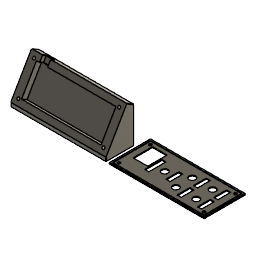
SoundRat (Autodesk Fusion 360 design; units mm, degrees)
Autodesk Fusion 360 part; units mm, degrees
sketch "Sketch1" plane through (0, 0, 0) normal (0, 0, 1) x (1, 0, 0)
  line L0 (74.95, -104) -> (175, -104)
  line L1 (175, -104) -> (175, -141.6)
  line L2 (175, -141.6) -> (74.95, -141.6)
  line L3 (74.95, -141.6) -> (74.95, -104)
  line L4 (67.45, -96.5) -> (182.5, -96.5)
  line L5 (182.5, -96.5) -> (182.5, -149.1)
  line L6 (182.5, -149.1) -> (67.45, -149.1)
  line L7 (67.45, -149.1) -> (67.45, -96.5)
  line L8 (67.45, -99) -> (64.95, -99)
  line L9 (64.95, -99) -> (64.95, -146.6)
  line L10 (64.95, -146.6) -> (67.45, -146.6)
  line L11 (67.45, -146.6) -> (67.45, -99)
  line L12 (182.5, -99) -> (185, -99)
  line L13 (185, -99) -> (185, -146.6)
  line L14 (185, -146.6) -> (182.5, -146.6)
  line L15 (182.5, -146.6) -> (182.5, -99)
  line L16 (78.95, -104) -> (88.95, -104)
  line L17 (88.95, -104) -> (88.95, -96.5)
  line L18 (88.95, -96.5) -> (78.95, -96.5)
  line L19 (78.95, -96.5) -> (78.95, -104)
  circle A0 centre (71.45, -103) radius 1.7
  circle A1 centre (71.45, -103) radius 3
  circle A2 centre (71.45, -142.6) radius 3
  circle A3 centre (71.45, -142.6) radius 1.7
  circle A4 centre (178.5, -103) radius 3
  circle A5 centre (178.5, -103) radius 1.7
  circle A6 centre (178.5, -142.6) radius 3
  circle A7 centre (178.5, -142.6) radius 1.7
  line L20 (182.5, -149.1) -> (185, -149.1)
  line L21 (185, -149.1) -> (185, -146.6)
  line L22 (185, -146.6) -> (182.5, -146.6)
  line L23 (182.5, -146.6) -> (182.5, -149.1)
  line L24 (185, -99) -> (182.5, -99)
  line L25 (182.5, -99) -> (182.5, -96.5)
  line L26 (182.5, -96.5) -> (185, -96.5)
  line L27 (185, -96.5) -> (185, -99)
  line L28 (67.45, -96.5) -> (64.95, -96.5)
  line L29 (64.95, -96.5) -> (64.95, -99)
  line L30 (64.95, -99) -> (67.45, -99)
  line L31 (67.45, -99) -> (67.45, -96.5)
  line L32 (67.45, -149.1) -> (64.95, -149.1)
  line L33 (64.95, -149.1) -> (64.95, -146.6)
  line L34 (64.95, -146.6) -> (67.45, -146.6)
  line L35 (67.45, -146.6) -> (67.45, -149.1)
  dimension "d1" = 100.05
  dimension "d2" = 37.6
  dimension "d3" = 7.5
  dimension "d4" = 7.5
  dimension "d5" = 7.5
  dimension "d6" = 7.5
  dimension "d7" = 2.5
  dimension "d8" = 2.5
  dimension "d9" = 2.5
  dimension "d10" = 2.5
  dimension "d11" = 2.5
  dimension "d12" = 2.5
  dimension "d19" = 4
  dimension "d20" = 10
  dimension "d26" = 3.4
  dimension "d29" = 6.5
  dimension "d30" = 4
  dimension "d31" = 6
  dimension "d32" = 3.4
  dimension "d33" = 6
  dimension "d34" = 6.5
  dimension "d35" = 4
  dimension "d36" = 3.4
  dimension "d37" = 6
  dimension "d38" = 3.4
  dimension "d39" = 6
  dimension "d40" = 6.5
  dimension "d41" = 4
  dimension "d42" = 4
  dimension "d43" = 6.5
  constraint horizontal L0
  constraint vertical L1
  constraint horizontal L2
  constraint vertical L3
  constraint horizontal L4
  constraint vertical L5
  constraint horizontal L6
  constraint vertical L7
  constraint horizontal L8
  constraint vertical L9
  constraint horizontal L10
  constraint vertical L11
  constraint coincident L7 L8.start
  constraint horizontal L12
  constraint vertical L13
  constraint horizontal L14
  constraint vertical L15
  constraint coincident L5 L12.start
  constraint horizontal L16
  constraint vertical L17
  constraint horizontal L18
  constraint vertical L19
  constraint coincident L4 L17.end
  constraint coincident L0 L16.start
  constraint concentric A0 A1
  constraint concentric A2 A3
  constraint concentric A4 A5
  constraint concentric A6 A7
  constraint horizontal L20
  constraint vertical L21
  constraint horizontal L22
  constraint vertical L23
  constraint horizontal L24
  constraint vertical L25
  constraint horizontal L26
  constraint vertical L27
  constraint horizontal L28
  constraint vertical L29
  constraint horizontal L30
  constraint vertical L31
  constraint horizontal L32
  constraint vertical L33
  constraint horizontal L34
  constraint vertical L35
  measures "d1" distance of L1 L3
  measures "d2" distance of L0 L2
  measures "d3" distance of L0 L4
  measures "d4" distance of L1 L5
  measures "d5" distance of L3 L7
  measures "d6" distance of L2 L6
  measures "d7" distance of L4 L8
  measures "d8" distance of L6 L10
  measures "d9" distance of L9 L11
  measures "d10" distance of L6 L14
  measures "d11" distance of L4 L12
  measures "d12" distance of L13 L15
  measures "d19" distance of L3 L19
  measures "d20" distance of L17 L19
  measures "d26" diameter of A0
  measures "d29" distance of L4 A0.centre
  measures "d30" distance of L7 A0.centre
  measures "d31" diameter of A1
  measures "d32" diameter of A3
  measures "d33" diameter of A2
  measures "d34" distance of L6 A2.centre
  measures "d35" distance of L7 A2.centre
  measures "d36" diameter of A5
  measures "d37" diameter of A4
  measures "d38" diameter of A7
  measures "d39" diameter of A6
  measures "d40" distance of L4 A4.centre
  measures "d41" distance of L15 A4.centre
  measures "d42" distance of L15 A6.centre
  measures "d43" distance of L6 A6.centre
sketch "Sketch3" plane through (0, 0, 0) normal (0, 0, 1) x (1, 0, 0)
  line L0 (181.1, -169) -> (183.6, -169)
  line L1 (181.1, -219.1) -> (66.05, -219.1)
  circle A0 centre (70.05, -212.6) radius 1.7
  line L2 (183.6, -169) -> (183.6, -216.6)
  line L3 (181.1, -166.5) -> (181.1, -219.1)
  line L4 (63.55, -216.6) -> (66.05, -216.6)
  line L5 (66.05, -216.6) -> (66.05, -169)
  line L6 (66.05, -219.1) -> (66.05, -166.5)
  line L7 (73.55, -174) -> (173.6, -174)
  line L8 (183.6, -216.6) -> (181.1, -216.6)
  line L9 (181.1, -216.6) -> (181.1, -169)
  circle A1 centre (70.05, -173) radius 1.7
  line L10 (63.55, -169) -> (63.55, -216.6)
  circle A2 centre (177.1, -173) radius 1.7
  circle A3 centre (177.1, -212.6) radius 1.7
  line L11 (88.45, -166.5) -> (79.45, -166.5)
  line L12 (73.55, -211.6) -> (73.55, -174)
  line L13 (173.6, -174) -> (173.6, -211.6)
  line L14 (66.05, -169) -> (63.55, -169)
  line L15 (66.05, -166.5) -> (181.1, -166.5)
  line L16 (173.6, -211.6) -> (73.55, -211.6)
  line L17 (79.45, -174) -> (88.45, -174)
  line L18 (93.5, -182.12) -> (98.5, -182.12)
  line L19 (98.5, -182.12) -> (98.5, -203.52)
  line L20 (98.5, -203.52) -> (93.5, -203.52)
  line L21 (93.5, -203.52) -> (93.5, -182.12)
  circle A4 centre (108.1, -193.12) radius 4
  line L22 (117.45, -184.87) -> (122.45, -184.87)
  line L23 (122.45, -184.87) -> (122.45, -200.77)
  line L24 (122.45, -200.77) -> (117.45, -200.77)
  line L25 (117.45, -200.77) -> (117.45, -184.87)
  circle A5 centre (132.45, -182.76) radius 4
  circle A6 centre (132.45, -203.45) radius 4
  line L26 (141.75, -174.5) -> (146.75, -174.5)
  line L27 (141.75, -190.5) -> (141.75, -174.5)
  line L28 (146.75, -190.5) -> (141.75, -190.5)
  line L29 (146.75, -174.5) -> (146.75, -190.5)
  line L30 (146.75, -195.1) -> (146.75, -211.1)
  line L31 (146.75, -211.1) -> (141.75, -211.1)
  line L32 (141.75, -211.1) -> (141.75, -195.1)
  line L33 (141.75, -195.1) -> (146.75, -195.1)
  circle A7 centre (158.1, -182.76) radius 4
  circle A8 centre (158.1, -203.45) radius 4
  line L34 (167.4, -211.1) -> (167.4, -195.1)
  line L35 (167.4, -195.1) -> (172.4, -195.1)
  line L36 (172.4, -195.1) -> (172.4, -211.1)
  line L37 (172.4, -211.1) -> (167.4, -211.1)
  line L38 (172.4, -190.5) -> (167.4, -190.5)
  line L39 (172.4, -174.5) -> (172.4, -190.5)
  line L40 (167.4, -174.5) -> (172.4, -174.5)
  line L41 (167.4, -190.5) -> (167.4, -174.5)
  line L42 (66.05, -169) -> (181.1, -169)
  line L43 (66.05, -216.6) -> (181.1, -216.6)
  line L44 (183.6, -169) -> (181.1, -169)
  line L45 (181.1, -169) -> (181.1, -166.5)
  line L46 (181.1, -166.5) -> (183.6, -166.5)
  line L47 (183.6, -166.5) -> (183.6, -169)
  line L48 (183.6, -216.6) -> (181.1, -216.6)
  line L49 (181.1, -216.6) -> (181.1, -219.1)
  line L50 (181.1, -219.1) -> (183.6, -219.1)
  line L51 (183.6, -219.1) -> (183.6, -216.6)
  line L52 (66.05, -219.1) -> (63.55, -219.1)
  line L53 (63.55, -219.1) -> (63.55, -216.6)
  line L54 (63.55, -216.6) -> (66.05, -216.6)
  line L55 (66.05, -216.6) -> (66.05, -219.1)
  line L56 (63.55, -169) -> (66.05, -169)
  line L57 (66.05, -169) -> (66.05, -166.5)
  line L58 (66.05, -166.5) -> (63.55, -166.5)
  line L59 (63.55, -166.5) -> (63.55, -169)
  dimension "d48" = 100.05
  dimension "d49" = 37.6
  dimension "d50" = 7.5
  dimension "d51" = 7.5
  dimension "d52" = 7.5
  dimension "d53" = 7.5
  dimension "d54" = 2.5
  dimension "d55" = 2.5
  dimension "d56" = 2.5
  dimension "d57" = 2.5
  dimension "d58" = 2.5
  dimension "d59" = 2.5
  dimension "d62" = 3.4
  dimension "d64" = 4
  dimension "d66" = 3.4
  dimension "d69" = 4
  dimension "d70" = 3.4
  dimension "d72" = 3.4
  dimension "d75" = 4
  dimension "d76" = 4
  dimension "d78" = 19.95
  dimension "d79" = 8.12
  dimension "d80" = 8.08
  dimension "d81" = 21.4
  dimension "d82" = 8
  dimension "d83" = 19.12
  dimension "d84" = 34.55
  dimension "d86" = 5
  dimension "d87" = 5
  dimension "d88" = 10.87
  dimension "d89" = 10.83
  dimension "d90" = 15.9
  dimension "d91" = 9.35
  dimension "d92" = 8
  dimension "d93" = 10
  dimension "d94" = 8.76
  dimension "d95" = 8
  dimension "d96" = 10
  dimension "d97" = 20.69
  dimension "d98" = 5
  dimension "d100" = 9.3
  dimension "d101" = 0.5
  dimension "d102" = 16
  dimension "d103" = 5
  dimension "d104" = 16
  dimension "d105" = 0.5
  dimension "d106" = 9.3
  dimension "d107" = 8
  dimension "d108" = 8
  dimension "d109" = 20.69
  dimension "d110" = 5
  dimension "d111" = 9.3
  dimension "d112" = 16
  dimension "d113" = 5
  dimension "d114" = 16
  dimension "d115" = 9.3
  dimension "d116" = 25.65
  dimension "d131" = 4
  dimension "d132" = 4
  dimension "d133" = 4
  dimension "d134" = 4
  constraint horizontal L7
  constraint vertical L13
  constraint horizontal L16
  constraint vertical L12
  constraint horizontal L15
  constraint vertical L3
  constraint horizontal L1
  constraint vertical L6
  constraint horizontal L14
  constraint vertical L10
  constraint horizontal L4
  constraint vertical L5
  constraint coincident L5.end L6
  constraint horizontal L0
  constraint vertical L2
  constraint horizontal L8
  constraint vertical L9
  constraint coincident L0.start L3
  constraint horizontal L17
  constraint horizontal L11
  constraint coincident L11.start L15
  constraint coincident L17.start L7
  constraint horizontal L18
  constraint vertical L19
  constraint horizontal L20
  constraint vertical L21
  constraint horizontal L22
  constraint vertical L23
  constraint horizontal L24
  constraint vertical L25
  constraint horizontal L26
  constraint vertical L29
  constraint horizontal L28
  constraint vertical L27
  constraint horizontal L33
  constraint vertical L30
  constraint horizontal L31
  constraint vertical L32
  constraint horizontal L40
  constraint vertical L39
  constraint horizontal L38
  constraint vertical L41
  constraint horizontal L35
  constraint vertical L36
  constraint horizontal L37
  constraint vertical L34
  constraint horizontal L44
  constraint vertical L45
  constraint horizontal L46
  constraint vertical L47
  constraint horizontal L48
  constraint vertical L49
  constraint horizontal L50
  constraint vertical L51
  constraint horizontal L52
  constraint vertical L53
  constraint horizontal L54
  constraint vertical L55
  constraint horizontal L56
  constraint vertical L57
  constraint horizontal L58
  constraint vertical L59
  measures "d48" distance of L12 L13
  measures "d49" distance of L7 L16
  measures "d50" distance of L7 L15
  measures "d51" distance of L3 L13
  measures "d52" distance of L6 L12
  measures "d53" distance of L1 L16
  measures "d54" distance of L14 L15
  measures "d55" distance of L1 L4
  measures "d56" distance of L5 L10
  measures "d57" distance of L1 L8
  measures "d58" distance of L0 L15
  measures "d59" distance of L2 L9
  measures "d62" diameter of A1
  measures "d64" distance of A1.centre L6
  measures "d66" diameter of A0
  measures "d69" distance of A0.centre L6
  measures "d70" diameter of A2
  measures "d72" diameter of A3
  measures "d75" distance of A2.centre L9
  measures "d76" distance of A3.centre L9
  measures "d78" distance of L12 L21
  measures "d79" distance of L7 L18
  measures "d80" distance of L16 L20
  measures "d81" distance of L18 L20
  measures "d82" diameter of A4
  measures "d83" distance of L7 A4.centre
  measures "d84" distance of L12 A4.centre
  measures "d86" distance of L19 L21
  measures "d87" distance of L23 L25
  measures "d88" distance of L7 L22
  measures "d89" distance of L16 L24
  measures "d90" distance of L22 L24
  measures "d91" distance of A4.centre L25
  measures "d92" diameter of A5
  measures "d93" distance of L23 A5.centre
  measures "d94" distance of L7 A5.centre
  measures "d95" diameter of A6
  measures "d96" distance of L23 A6.centre
  measures "d97" distance of A5.centre A6.centre
  measures "d98" distance of L27 L29
  measures "d100" distance of A5.centre L27
  measures "d101" distance of L7 L26
  measures "d102" distance of L26 L28
  measures "d103" distance of L30 L32
  measures "d104" distance of L31 L33
  measures "d105" distance of L16 L31
  measures "d106" distance of A6.centre L32
  measures "d107" diameter of A7
  measures "d108" diameter of A8
  measures "d109" distance of A8.centre A7.centre
  measures "d110" distance of L39 L41
  measures "d111" distance of A7.centre L41
  measures "d112" distance of L38 L40
  measures "d113" distance of L34 L36
  measures "d114" distance of L35 L37
  measures "d115" distance of A8.centre L34
  measures "d116" distance of A5.centre A7.centre
  measures "d131" distance of A1.centre L42
  measures "d132" distance of A2.centre L42
  measures "d133" distance of A0.centre L43
  measures "d134" distance of A3.centre L43
move_body "Move1" [no effect]
move_body "Move2" [no effect]
move_body "Move3" [no effect]
move_body "Move4" [no effect]
move_body "Move5" [no effect]
extrude "Extrude16" add sketch "Sketch1" along normal blind 2.5 contours L0 L1 L2 L3 L16 makes body 1
extrude "Extrude17" add sketch "Sketch1" along normal blind 10.4 contours L0 L1 L2 L3 L4 L5 L6 L7 L11 L15 L17 L19 L23 L25 L31 L35 | L0 L4 L16 L17 L18 L19 | L7 L8 L28 L29 L30 L31 | L5 L12 L24 L25 L26 L27 | L7 L8 L9 L10 L11 L30 L34 | L5 L12 L13 L14 L15 L22 L24 | L7 L10 L32 L33 L34 L35 | L5 L14 L20 L21 L22 L23 | A0 | A1 | A2 | A3 | A4 | A5 | A6 | A7 bodies 1
extrude "Extrude18" cut sketch "Sketch1" along normal blind 6 from surface at 5 contours L0 L4 L16 L17 L18 L19 bodies 1
extrude "Extrude19" cut sketch "Sketch1" along normal blind 3.1 contours A1 | A2 | A4 | A6 bodies 1
extrude "Extrude20" cut sketch "Sketch1" along normal blind 10.4 contours A0 | A3 | A5 | A7 bodies 1
move_body "Move6" bodies 1 to x (1, 0, 0) y (0, 0.5, 0.866025) z (0, -0.866025, 0.5) at (0, -74.55, 129.1244)
sketch "Sketch7" plane through (64.95, 0, 0) normal (-1, 0, 0) x (0, -1, 0)
  line L0 (122.8, 45.5529) -> (149.1, 0)
  line L1 (149.1, 0) -> (158.1067, 5.2)
  line L2 (158.1067, 5.2) -> (131.8067, 50.7529)
  line L3 (131.8067, 50.7529) -> (122.8, 45.5529)
  line L4 (122.8, 45.5529) -> (122.8, 0)
  line L5 (122.8, 0) -> (149.1, 0)
  line L6 (158.1067, 5.2) -> (158.1067, 0)
  line L7 (158.1067, 0) -> (149.1, 0)
  constraint coincident L0.start L3.end
  constraint vertical L4
  constraint coincident L0.end L1.start
  constraint perpendicular L4 L5
  constraint coincident L1.end L2.start
  constraint vertical L6
  constraint perpendicular L6 L7
extrude "Extrude21" add sketch "Sketch7" against normal blind 120 contours L0 L4 L5 | L1 L6 L7 bodies 1
extrude "Extrude22" add 1 faces at (184.95, -131.5667, 15.1843) along direction (1, 0, 0) blind 0.05 on bodies 1 bodies 1
extrude "Extrude23" add 1 faces at (184.95, -155.1044, 1.7333) along direction (1, 0, 0) blind 0.05 on bodies 1 bodies 1
extrude "Extrude24" cut 4 faces at (177.7558, -125.7844, 40.3837) (179.2219, -145.5844, 6.0891) (71.8404, -126.4322, 39.2618) (72.1281, -145.0948, 6.9373) along direction (0, 0.866025, -0.5) blind 40 on bodies 1 bodies 1
extrude "Extrude26" add sketch "Sketch3" along normal blind 1 separate body contours L3 L5 L6 L9 L42 L43 | A0 | L7 L12 L13 L16 L17 | A1 | A2 | A3 makes body 2
extrude "Extrude27" add sketch "Sketch3" along normal blind 1.2 separate body contours L0 L3 L44 L45 L46 L47 | L3 L6 L11 L15 L42 L45 L57 | L0 L2 L3 L8 L9 L44 L48 | L1 L3 L6 L43 L49 L55 | L6 L14 L56 L57 L58 L59 | L4 L5 L6 L10 L14 L54 L56 | L4 L6 L52 L53 L54 L55 makes body 3
extrude "Extrude28" add sketch "Sketch3" along normal blind 1.2 contours L3 L8 L48 L49 L50 L51 bodies 2 3
extrude "Extrude29" add 1 faces at (104.4, -218.2667, 1.2) along direction (0, 0, 1) blind 0.2 on bodies 2 bodies 2
chamfer "Chamfer4" distance 0.5 angle 45 8 edges at (63.55, -192.8, 1.4) (123.575, -166.5, 1.4) (183.6, -192.8, 1.4) (123.575, -219.1, 1.4) (63.55, -219.1, 0.7) (183.6, -219.1, 0.7) (183.6, -166.5, 0.7) (63.55, -166.5, 0.7) on bodies 2
extrude "Extrude30" cut sketch "Sketch3" along normal blind 2 contours A0 | A1 | A2 | A3 bodies 2
chamfer "Chamfer5" distance 0.5 angle 45 2 edges at (83.95, -127.1301, 48.0529) (83.95, -130.8801, 41.5577) on bodies 1
chamfer "Chamfer6" distance 0.5 angle 45 11 edges at (124.975, -158.1067, 0) (64.95, -158.1067, 2.6) (185, -158.1067, 2.6) (185, -140.4533, 0) (185, -122.8, 22.7765) (124.975, -122.8, 0) (124.975, -122.8, 45.5529) (185, -127.3033, 48.1529) (64.95, -127.3033, 48.1529) (64.95, -122.8, 22.7765) (64.95, -140.4533, 0) on bodies 1
chamfer "Chamfer7" distance 0.5 angle 45 2 edges at (88.95, -129.2519, 49.2779) (78.95, -129.2519, 49.2779) on bodies 1
chamfer "Chamfer8" distance 0.5 angle 45 2 edges at (78.95, -133.0019, 42.7827) (88.95, -133.0019, 42.7827) on bodies 1
move_body "Move7" bodies 2 to x (1, 0, 0) y (0, 0.5, 0.866025) z (0, -0.866025, 0.5) at (1.3343, -48.7637, 195.0311)
move_body "Move8" bodies 2 to x (1, 0, 0) y (0, 1, 0) z (0, 0, 1) at (0.1947, 0.0649, 0.1124)
sketch "Sketch8" plane through (0, -121.8898, 70.3731) normal (0, -0.866025, 0.5) x (1, 0, 0)
  circle A0 centre (71.579, -67.9501) radius 1.7
  circle A1 centre (178.629, -67.9501) radius 1.7
  circle A2 centre (71.579, -28.3501) radius 1.7
  circle A3 centre (178.629, -28.3501) radius 1.7
  circle A4 centre (133.979, -58.8001) radius 4
  line L0 (143.279, -66.4501) -> (143.279, -50.4501)
  line L1 (143.279, -50.4501) -> (148.279, -50.4501)
  line L2 (148.279, -50.4501) -> (148.279, -66.4501)
  line L3 (148.279, -66.4501) -> (143.279, -66.4501)
  line L4 (123.979, -56.1201) -> (118.979, -56.1201)
  line L5 (118.979, -56.1201) -> (118.979, -40.2201)
  line L6 (118.979, -40.2201) -> (123.979, -40.2201)
  line L7 (123.979, -40.2201) -> (123.979, -56.1201)
  circle A5 centre (133.979, -38.1101) radius 4
  line L8 (100.029, -58.8701) -> (95.029, -58.8701)
  line L9 (95.029, -58.8701) -> (95.029, -37.4701)
  line L10 (95.029, -37.4701) -> (100.029, -37.4701)
  line L11 (100.029, -37.4701) -> (100.029, -58.8701)
  line L12 (143.279, -29.8501) -> (148.279, -29.8501)
  line L13 (148.279, -29.8501) -> (148.279, -45.8501)
  line L14 (148.279, -45.8501) -> (143.279, -45.8501)
  line L15 (143.279, -45.8501) -> (143.279, -29.8501)
  circle A6 centre (109.629, -48.4701) radius 4
  line L16 (173.929, -50.4501) -> (173.929, -66.4501)
  line L17 (173.929, -66.4501) -> (168.929, -66.4501)
  line L18 (168.929, -66.4501) -> (168.929, -50.4501)
  line L19 (168.929, -50.4501) -> (173.929, -50.4501)
  circle A7 centre (159.629, -38.1101) radius 4
  circle A8 centre (159.629, -58.8001) radius 4
  line L20 (173.929, -45.8501) -> (168.929, -45.8501)
  line L21 (168.929, -45.8501) -> (168.929, -29.8501)
  line L22 (168.929, -29.8501) -> (173.929, -29.8501)
  line L23 (173.929, -29.8501) -> (173.929, -45.8501)
  line L24 (67.579, -24.3501) -> (67.579, -71.9501)
  line L25 (67.579, -71.9501) -> (182.629, -71.9501)
  line L26 (182.629, -71.9501) -> (182.629, -24.3501)
  line L27 (182.629, -24.3501) -> (67.579, -24.3501)
  line L28 (75.079, -53.5201) -> (93.2419, -53.5201)
  line L29 (93.2419, -53.5201) -> (93.2419, -29.3501)
  line L30 (93.2419, -29.3501) -> (75.079, -29.3501)
  line L31 (75.079, -29.3501) -> (75.079, -53.5201)
  dimension "d176" = 5
  dimension "d177" = 7.5
  constraint horizontal L28
  constraint vertical L29
  constraint horizontal L30
  constraint vertical L31
  measures "d176" distance of L27 L30
  measures "d177" distance of L24 L31
extrude "Extrude31" cut sketch "Sketch8" against normal blind 2 contours L28 L29 L30 L31 bodies 2
move_body "Move9" bodies 2 to x (1, 0, 0) y (0, 0.5, -0.866025) z (0, 0.866025, 0.5) at (124, -84.2799, -135.1823)
move_body "Move10" bodies 2 to x (1, 0, 0) y (0, 1, 0) z (0, 0, 1) at (0, 0, -4)
equation "d1 = 99.95 mm + 0.1 mm"
equation "d2 = 37.5 mm + 0.1 mm"
equation "d29 = 4 mm + 2.5 mm"
equation "d34 = 4 mm + 2.5 mm"
equation "d40 = 4 mm + 2.5 mm"
equation "d43 = 4.00 mm + 2.5 mm"
equation "d48 = 99.95 mm + 0.1 mm"
equation "d49 = 37.5 mm + 0.1 mm"
equation "d78 = 19.85 mm + 0.1 mm"
equation "d79 = 8.02 mm + 0.1 mm"
equation "d80 = 7.98 mm + 0.1 mm"
equation "d83 = 19.02 mm + 0.1 mm"
equation "d84 = 34.45 mm + 0.1 mm"
equation "d88 = 10.77 mm + 0.1 mm"
equation "d89 = 10.73 mm + 0.1 mm"
equation "d94 = 8.66 mm + 0.1 mm"
equation "d101 = 0.4 mm + 0.1 mm"
equation "d105 = 0.4 mm + 0.1 mm"
equation "d176 = 7.5 mm - 2.5 mm"
equation "d177 = 10 mm - 2.5 mm"
